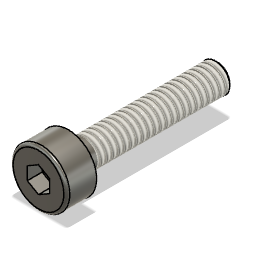
fusion_export (Autodesk Fusion 360 archive; units mm, degrees)
design "Innensechskantschraube DIN EN ISO 4762 - M2 x 10 Stahl 4.6 Einfach"
description: Innensechskantschraube DIN EN ISO 4762 - M2 x 10
Autodesk Fusion 360 part; units mm, degrees
sketch "Sketch1" plane through (0, 0, 0) normal (0, 1, 0) x (1, 0, 0)
  line L0 (-1, 0) -> (-1, 10)
  line L1 (-1, 10) -> (0, 10)
  line L2 (0, 10) -> (0, -2)
  line L3 (-1, 0) -> (-1.9, 0)
  line L4 (-1.9, 0) -> (-1.9, -2)
  line L5 (-1.9, -2) -> (0, -2)
  dimension "d9" = 2
  dimension "d66" = 3.8
  dimension "d68" = 10
  dimension "d79" = 2
  constraint perpendicular L0 L1
  constraint collinear origin L1.end L2.end
  constraint perpendicular L0 L3
  constraint coincident origin L3
  constraint vertical L0
  constraint vertical L2
  constraint parallel L2 L4
  constraint coincident L2 L5.end
  constraint perpendicular L2 L5
  measures "d68" distance of origin L1.end
  measures "d79" distance of L3.end L4.end
revolve "Revolve1" add sketch "Sketch1" angle 360 about axis through (0, 0, -10) along (0, 0, 1)
ref_plane "WorkPlane1" through (0, 0, 2) normal (0, 0, 1) x (1, 0, 0)
sketch "Sketch6" plane through (0, 0, 2) normal (0, 0, 1) x (1, 0, 0)
  line L0 (-0.75, 0) -> (0.75, 0) construction
  line L1 (0, 0) -> (-0.75, 0.433)
  line L2 (-0.75, -0.433) -> (-0.75, 0.433)
  line L3 (-0.75, -0.433) -> (0, 0)
  dimension "d72" = 1.5
  dimension "d104" = 150
  constraint horizontal L0
  constraint midpoint L1.start L0
  constraint coincident L1.start L3.end
  constraint perpendicular L0 L2
  constraint midpoint L0.start L2
  constraint coincident L1.end L2.end
  measures "d72" distance of L0.start L0.end
  measures "d104" angle of L0 L1
extrude "Extrude1" cut sketch "Sketch6" against normal blind 1
pattern_circular "C-Pattern1" count 6 over 360 about axis through (0, 0, 1.75) along (0, 0, 1) of "Extrude1"
extrude "Extrude2" cut 1 faces at (-0.25, -0.1443, 1) along direction (0, 0, -1) blind 1 draft -85
fillet "Fillet4" radius 0.2 1 edges at (-1.7714, 0.6871, 2)
thread "Thread2" "ISO Metric profile 2.0 M2x0.4 6g" major diameter 1.9335 minor diameter 1.478 pitch 0.4 angle 60 resizes the face on face at (-0.995, 0.0996, -3.3333) from (0, 0, -1) to (0, 0, -10)
sketch "Sketch7" plane through (0, 0, 0) normal (0, 1, 0) x (1, 0, 0)
  line L0 (-1.02, 10) -> (-1.02, 9.8)
  line L1 (-1.02, 9.8) -> (-0.82, 10)
  line L2 (0, 10) -> (0, -2)
  line L3 (-1.02, 10) -> (0, 10)
  dimension "d99" = 1.02
  dimension "d101" = 45
  dimension "d103" = 0.2
  constraint coincident L2.start L3.end
  constraint perpendicular L2 L3
  constraint coincident L1.end L3
  constraint perpendicular L0 L3
  measures "d99" distance of origin L0
  measures "d101" angle of L0 L1
  measures "d103" vertical distance of L0.end L1.end
revolve "Revolve3" cut sketch "Sketch7" angle 360 about axis through (0, 0, 1.75) along (0, 0, 1)
equation "d9 = adsk_nomdia"
equation "adsk_nomlen = 10.00 mm"
equation "adsk_headh = 2.00 mm"
equation "adsk_headdia = 3.80 mm"
equation "adsk_nomdia = 2.00 mm"
equation "adsk_philwidth = 1.50 mm"
equation "d31 = -adsk_phildepth"
equation "adsk_phildepth = 1.00 mm"
equation "d66 = adsk_headdia"
equation "d68 = adsk_nomlen"
equation "d71 = adsk_headh"
equation "d72 = adsk_philwidth"
equation "d76 = -adsk_phildepth"
equation "d79 = adsk_headh"
equation "adsk_thrlen = 9.00 mm"
equation "d84 = adsk_thrlen"
equation "d86 = adsk_nomdia * 0.1"
equation "d99 = adsk_nomdia * 0.51"
equation "adsk_startang = 45.00 deg"
equation "d101 = adsk_startang"
equation "adsk_pitch1 = 0.40 mm"
equation "d103 = adsk_startlen"
equation "adsk_startlen = 0.20 mm"

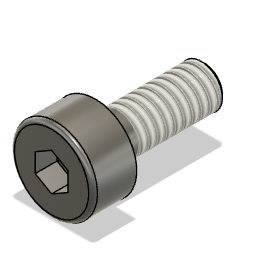
design "Innensechskantschraube DIN EN ISO 4762 - M2 x 5 Stahl 4.6 Einfach"
description: Innensechskantschraube DIN EN ISO 4762 - M2 x 5
Autodesk Fusion 360 part; units mm, degrees
sketch "Sketch1" plane through (0, 0, 0) normal (0, 1, 0) x (1, 0, 0)
  line L0 (-1, 0) -> (-1, 5)
  line L1 (-1, 5) -> (0, 5)
  line L2 (0, 5) -> (0, -2)
  line L3 (-1, 0) -> (-1.9, 0)
  line L4 (-1.9, 0) -> (-1.9, -2)
  line L5 (-1.9, -2) -> (0, -2)
  dimension "d9" = 2
  dimension "d66" = 3.8
  dimension "d68" = 5
  dimension "d79" = 2
  constraint perpendicular L0 L1
  constraint collinear origin L1.end L2.end
  constraint perpendicular L0 L3
  constraint coincident origin L3
  constraint vertical L0
  constraint vertical L2
  constraint parallel L2 L4
  constraint coincident L2 L5.end
  constraint perpendicular L2 L5
  measures "d68" distance of origin L1.end
  measures "d79" distance of L3.end L4.end
revolve "Revolve1" add sketch "Sketch1" angle 360 about axis through (0, 0, -5) along (0, 0, 1)
ref_plane "WorkPlane1" through (0, 0, 2) normal (0, 0, 1) x (1, 0, 0)
sketch "Sketch6" plane through (0, 0, 2) normal (0, 0, 1) x (1, 0, 0)
  line L0 (-0.75, 0) -> (0.75, 0) construction
  line L1 (0, 0) -> (-0.75, 0.433)
  line L2 (-0.75, -0.433) -> (-0.75, 0.433)
  line L3 (-0.75, -0.433) -> (0, 0)
  dimension "d72" = 1.5
  dimension "d104" = 150
  constraint horizontal L0
  constraint midpoint L1.start L0
  constraint coincident L1.start L3.end
  constraint perpendicular L0 L2
  constraint midpoint L0.start L2
  constraint coincident L1.end L2.end
  measures "d72" distance of L0.start L0.end
  measures "d104" angle of L0 L1
extrude "Extrude1" cut sketch "Sketch6" against normal blind 1
pattern_circular "C-Pattern1" count 6 over 360 about axis through (0, 0, 1.75) along (0, 0, 1) of "Extrude1"
extrude "Extrude2" cut 1 faces at (-0.25, -0.1443, 1) along direction (0, 0, -1) blind 1 draft -85
fillet "Fillet4" radius 0.2 1 edges at (-1.7714, 0.6871, 2)
thread "Thread2" "ISO Metric profile 2.0 M2x0.4 6g" major diameter 1.9335 minor diameter 1.478 pitch 0.4 angle 60 resizes the face on face at (-0.995, 0.0996, -1.6667) from (0, 0, -1) to (0, 0, -5)
sketch "Sketch7" plane through (0, 0, 0) normal (0, 1, 0) x (1, 0, 0)
  line L0 (-1.02, 5) -> (-1.02, 4.8)
  line L1 (-1.02, 4.8) -> (-0.82, 5)
  line L2 (0, 5) -> (0, -2)
  line L3 (-1.02, 5) -> (0, 5)
  dimension "d99" = 1.02
  dimension "d101" = 45
  dimension "d103" = 0.2
  constraint coincident L2.start L3.end
  constraint perpendicular L2 L3
  constraint coincident L1.end L3
  constraint perpendicular L0 L3
  measures "d99" distance of origin L0
  measures "d101" angle of L0 L1
  measures "d103" vertical distance of L0.end L1.end
revolve "Revolve3" cut sketch "Sketch7" angle 360 about axis through (0, 0, 1.75) along (0, 0, 1)
equation "d9 = adsk_nomdia"
equation "adsk_nomlen = 5.00 mm"
equation "adsk_headh = 2.00 mm"
equation "adsk_headdia = 3.80 mm"
equation "adsk_nomdia = 2.00 mm"
equation "adsk_philwidth = 1.50 mm"
equation "d31 = -adsk_phildepth"
equation "adsk_phildepth = 1.00 mm"
equation "d66 = adsk_headdia"
equation "d68 = adsk_nomlen"
equation "d71 = adsk_headh"
equation "d72 = adsk_philwidth"
equation "d76 = -adsk_phildepth"
equation "d79 = adsk_headh"
equation "adsk_thrlen = 4.00 mm"
equation "d84 = adsk_thrlen"
equation "d86 = adsk_nomdia * 0.1"
equation "d99 = adsk_nomdia * 0.51"
equation "adsk_startang = 45.00 deg"
equation "d101 = adsk_startang"
equation "adsk_pitch1 = 0.40 mm"
equation "d103 = adsk_startlen"
equation "adsk_startlen = 0.20 mm"
